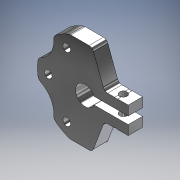
# Autodesk Inventor part: オムニ固定する
Saved by Autodesk Inventor 2019.4 (Build 234330000, 330)
## iProperties
Created: 2021-08-30
Part Number: オムニ固定する
Material: アルミニウム 6061
Document SubType Name: Modeling
Designer: 堀川皓史
Density: 2.7 g/cm^3
Appearance: アルミニウム - フラット
Author: 堀川皓史
Autodesk Inventor part; units mm, degrees
ref_plane "YZ Plane" through (0, 0, 0) normal (1, 0, 0) x (0, 1, 0)
ref_plane "XZ Plane" through (0, 0, 0) normal (0, 1, 0) x (-1, 0, 0)
ref_plane "XY Plane" through (0, 0, 0) normal (0, 0, 1) x (1, 0, 0)
sketch "スケッチ1" plane through (0, 0, 0) normal (0, 0, 1) x (1, 0, 0)
  arc A0 (3.7417, 1.55) -> (3.7417, -1.55) centre (0, 0) ccw
  circle A1 centre (-15.5, 0) radius 1.6
  circle A2 centre (-7.75, 13.4234) radius 1.6
  circle A3 centre (-7.75, -13.4234) radius 1.6
  line L0 (-7.75, 13.4234) -> (0, 0) construction
  line L1 (0, 0) -> (-7.75, -13.4234) construction
  line L2 (-15.5, 0) -> (0, 0) construction
  arc A4 (-6.3339, 18.9706) -> (-13.2621, 14.9706) centre (0, 0) ccw
  arc A5 (-19.5959, 4) -> (-19.5959, -4) centre (0, 0) ccw
  arc A6 (-13.2621, -14.9706) -> (-6.3339, -18.9706) centre (0, 0) ccw
  arc A7 (-19.5959, 4) -> (-13.2621, 14.9706) centre (-23.1306, 13.3545) ccw
  line L3 (-6.3339, 18.9706) -> (-7.75, 13.4234) construction
  line L4 (-13.2621, 14.9706) -> (-7.75, 13.4234) construction
  line L5 (-13.2621, 14.9706) -> (-6.3339, 18.9706) construction
  line L6 (-19.5959, 4) -> (-15.5, 0) construction
  line L7 (-15.5, 0) -> (-19.5959, -4) construction
  line L8 (-19.5959, -4) -> (-19.5959, 4) construction
  line L9 (-13.2621, -14.9706) -> (-6.3339, -18.9706) construction
  line L10 (-6.3339, -18.9706) -> (-7.75, -13.4234) construction
  line L11 (-7.75, -13.4234) -> (-13.2621, -14.9706) construction
  arc A8 (-13.2621, -14.9706) -> (-19.5959, -4) centre (-23.1306, -13.3545) ccw
  line L12 (8, 5.55) -> (12.3462, 5.55)
  line L13 (18, 5.55) -> (18, 1.55)
  line L14 (18, 1.55) -> (3.7417, 1.55)
  line L15 (3.7417, -1.55) -> (18, -1.55)
  line L16 (18, -1.55) -> (18, -5.55)
  line L17 (18, -5.55) -> (13.6538, -5.55)
  line L18 (-6.3339, 18.9706) -> (3, 18.9706)
  line L19 (3, 18.9706) -> (8, 5.55)
  line L20 (-6.3339, -18.9706) -> (3, -18.9706)
  line L21 (3, -18.9706) -> (8, -5.55)
  arc A9 (12.3462, 5.55) -> (13.6538, 5.55) centre (13, 6.9) ccw
  arc A10 (13.6538, -5.55) -> (12.3462, -5.55) centre (13, -6.9) ccw
  arc A11 (13.6538, 5.55) -> (12.3462, 5.55) centre (13, 6.9) ccw construction
  arc A12 (12.3462, -5.55) -> (13.6538, -5.55) centre (13, -6.9) ccw construction
  line L22 (13.6538, 5.55) -> (18, 5.55)
  line L23 (12.3462, 5.55) -> (13.6538, 5.55) construction
  line L24 (13.6538, -5.55) -> (12.3462, -5.55) construction
  line L25 (12.3462, -5.55) -> (8, -5.55)
  dimension "d18" = 8.1
  dimension "d24" = 3.2
  dimension "d25" = 3.2
  dimension "d26" = 60
  dimension "d27" = 60
  dimension "d28" = 15.5
  dimension "d29" = 3.2
  dimension "d30" = 20
  dimension "d31" = 20
  dimension "d36" = 3.1
  dimension "d37" = 1.55
  dimension "d38" = 4
  dimension "d39" = 4
  dimension "d40" = 10
  dimension "d44" = 18
  dimension "d45" = 18
  dimension "d47" = 3
  dimension "d48" = 1.35
  dimension "d49" = 3
  dimension "d50" = 1.35
  dimension "d51" = 5
  dimension "d59" = 10
  dimension "d60" = 10
  dimension "d61" = 8
  dimension "d62" = 8
  dimension "d63" = 8
  dimension "d64" = 5
  constraints: 52 end point, 20 point on circle, 13 centre point, 8 horizontal, 7 perpendicular, 4 coincident, 4 equal length, 4 vertical alignment, 1 concentric, 1 point on line
  measures "d18" diameter of A0
  measures "d24" diameter of A2
  measures "d25" diameter of A3
  measures "d26" angle of L2 L0
  measures "d27" angle of L1 L2
  measures "d28" distance of L2.start L0.end
  measures "d29" diameter of A1
  measures "d30" radius of A4
  measures "d31" radius of A5
  measures "d36" distance between parallel lines of L15 L14
  measures "d37" distance from line of point (0, 0) L14
  measures "d38" distance between parallel lines of L14 L12
  measures "d39" distance between parallel lines of L17 L15
  measures "d40" distance of L16.end L21.end
  measures "d44" distance from line of L16 point (0, 0)
  measures "d45" distance from line of L13 point (0, 0)
  measures "d47" diameter of A9
  measures "d48" distance from line of L12 A9.centre
  measures "d49" diameter of A10
  measures "d50" distance from line of A10.centre L17
  measures "d51" distance from line of L13 A9.centre
  measures "d59" radius of A7
  measures "d60" radius of A8
  measures "d61" distance of L7.end L6.start
  measures "d62" distance of L4.start L3.start
  measures "d63" distance of L9.start L9.end
  measures "d64" horizontal distance of L18.end L12.start
extrude "押し出し1" add sketch "スケッチ1" along normal blind 6
sketch "スケッチ2" plane through (13.6538, 5.55, 0) normal (0, 1, 0) x (1, 0, 0)
  circle A0 centre (-0.6538, -3) radius 1.6
  line L0 (0, 0) -> (-1.3077, 0) projected
  point P0 (-13.6538, 0)
  point P1 (-0.6538, 0)
  dimension "d54" = 3.2
  dimension "d55" = 3
  constraints: 1 centre point, 1 midpoint, 1 vertical alignment
  measures "d54" diameter of A0
  measures "d55" distance from line of L0 A0.centre
extrude "押し出し2" cut sketch "スケッチ2" against normal through all
fillet "フィレット1" radius 2 10 edges at (8, 5.55, 3) (3, 18.9706, 3) (-6.3339, 18.9706, 3) (-13.2621, 14.9706, 3) (-19.5959, 4, 3) (-19.5959, -4, 3) (-13.2621, -14.9706, 3) (-6.3339, -18.9706, 3) (3, -18.9706, 3) (8, -5.55, 3)
equation "\"d45\" = d44"
